box test cut_v2 (Autodesk Fusion 360 design; units mm, degrees)
Autodesk Fusion 360 part; units mm, degrees
note: some values were not read from the file. Set by a fixed rule: which sketch regions a step uses.
sketch "test" plane through (0, 0, 0) normal (0, 0, 1) x (1, 0, 0)
sketch "test (1)" plane through (0, 0, 0) normal (0, 0, 1) x (1, 0, 0)
  line L0 (0, 0) -> (0, 15.1)
  line L1 (0, 15.1) -> (3.175, 15.1)
  line L2 (3.175, 15.1) -> (3.175, 24.9)
  line L3 (3.175, 24.9) -> (0, 24.9)
  line L4 (0, 24.9) -> (0, 35.1)
  line L5 (0, 35.1) -> (3.175, 35.1)
  line L6 (3.175, 35.1) -> (3.175, 44.9)
  line L7 (3.175, 44.9) -> (0, 44.9)
  line L8 (0, 44.9) -> (0, 55.1)
  line L9 (0, 55.1) -> (3.175, 55.1)
  line L10 (3.175, 55.1) -> (3.175, 64.9)
  line L11 (3.175, 64.9) -> (0, 64.9)
  line L12 (0, 64.9) -> (0, 75.1)
  line L13 (0, 75.1) -> (3.175, 75.1)
  line L14 (3.175, 75.1) -> (3.175, 84.9)
  line L15 (3.175, 84.9) -> (0, 84.9)
  line L16 (0, 84.9) -> (0, 95.1)
  line L17 (0, 95.1) -> (3.175, 95.1)
  line L18 (3.175, 95.1) -> (3.175, 104.9)
  line L19 (3.175, 104.9) -> (0, 104.9)
  line L20 (0, 104.9) -> (0, 120)
  circle A0 centre (2.3644, 15.6906) radius 1.005
  circle A1 centre (2.3644, 24.3094) radius 1.005
  circle A2 centre (2.3644, 35.6906) radius 1.005
  circle A3 centre (2.3644, 44.3094) radius 1.005
  circle A4 centre (2.3644, 55.6906) radius 1.005
  circle A5 centre (2.3644, 64.3094) radius 1.005
  circle A6 centre (2.3644, 75.6906) radius 1.005
  circle A7 centre (2.3644, 84.3094) radius 1.005
  circle A8 centre (2.3644, 95.6906) radius 1.005
  circle A9 centre (2.3644, 104.3094) radius 1.005
  line L21 (-5.185, 0) -> (-5.185, 14.9)
  line L22 (-5.185, 14.9) -> (-2.01, 14.9)
  line L23 (-2.01, 14.9) -> (-2.01, 25.1)
  line L24 (-2.01, 25.1) -> (-5.185, 25.1)
  line L25 (-5.185, 25.1) -> (-5.185, 34.9)
  line L26 (-5.185, 34.9) -> (-2.01, 34.9)
  line L27 (-2.01, 34.9) -> (-2.01, 45.1)
  line L28 (-2.01, 45.1) -> (-5.185, 45.1)
  line L29 (-5.185, 45.1) -> (-5.185, 54.9)
  line L30 (-5.185, 54.9) -> (-2.01, 54.9)
  line L31 (-2.01, 54.9) -> (-2.01, 65.1)
  line L32 (-2.01, 65.1) -> (-5.185, 65.1)
  line L33 (-5.185, 65.1) -> (-5.185, 74.9)
  line L34 (-5.185, 74.9) -> (-2.01, 74.9)
  line L35 (-2.01, 74.9) -> (-2.01, 85.1)
  line L36 (-2.01, 85.1) -> (-5.185, 85.1)
  line L37 (-5.185, 85.1) -> (-5.185, 94.9)
  line L38 (-5.185, 94.9) -> (-2.01, 94.9)
  line L39 (-2.01, 94.9) -> (-2.01, 105.1)
  line L40 (-2.01, 105.1) -> (-5.185, 105.1)
  line L41 (-5.185, 105.1) -> (-5.185, 120)
  circle A10 centre (-4.3744, 14.3094) radius 1.005
  circle A11 centre (-4.3744, 25.6906) radius 1.005
  circle A12 centre (-4.3744, 34.3094) radius 1.005
  circle A13 centre (-4.3744, 45.6906) radius 1.005
  circle A14 centre (-4.3744, 54.3094) radius 1.005
  circle A15 centre (-4.3744, 65.6906) radius 1.005
  circle A16 centre (-4.3744, 74.3094) radius 1.005
  circle A17 centre (-4.3744, 85.6906) radius 1.005
  circle A18 centre (-4.3744, 94.3094) radius 1.005
  circle A19 centre (-4.3744, 105.6906) radius 1.005
  line L42 (0, 0) -> (-5.185, 0)
  line L43 (0, 120) -> (-5.185, 120)
  dimension "d13" = 15.1
  dimension "d14" = 3.175
  dimension "d15" = 9.8
  dimension "d16" = 3.175
  dimension "d17" = 10.2
  dimension "d18" = 3.175
  dimension "d19" = 9.8
  dimension "d20" = 3.175
  dimension "d21" = 10.2
  dimension "d22" = 3.175
  dimension "d23" = 9.8
  dimension "d24" = 3.175
  dimension "d25" = 10.2
  dimension "d26" = 3.175
  dimension "d27" = 9.8
  dimension "d28" = 3.175
  dimension "d29" = 10.2
  dimension "d30" = 3.175
  dimension "d31" = 9.8
  dimension "d32" = 3.175
  dimension "d33" = 15.1
  dimension "d34" = 2.01
  dimension "d35" = 2.01
  dimension "d36" = 2.01
  dimension "d37" = 2.01
  dimension "d38" = 2.01
  dimension "d39" = 2.01
  dimension "d40" = 2.01
  dimension "d41" = 2.01
  dimension "d42" = 2.01
  dimension "d43" = 2.01
  dimension "d44" = 14.9
  dimension "d45" = 3.175
  dimension "d46" = 10.2
  dimension "d47" = 3.175
  dimension "d48" = 9.8
  dimension "d49" = 3.175
  dimension "d50" = 10.2
  dimension "d51" = 3.175
  dimension "d52" = 9.8
  dimension "d53" = 3.175
  dimension "d54" = 10.2
  dimension "d55" = 3.175
  dimension "d56" = 9.8
  dimension "d57" = 3.175
  dimension "d58" = 10.2
  dimension "d59" = 3.175
  dimension "d60" = 9.8
  dimension "d61" = 3.175
  dimension "d62" = 10.2
  dimension "d63" = 3.175
  dimension "d64" = 14.9
  dimension "d65" = 2.01
  dimension "d66" = 2.01
  dimension "d67" = 2.01
  dimension "d68" = 2.01
  dimension "d69" = 2.01
  dimension "d70" = 2.01
  dimension "d71" = 2.01
  dimension "d72" = 2.01
  dimension "d73" = 2.01
  dimension "d74" = 2.01
  constraint vertical L0
  constraint horizontal L1
  constraint vertical L2
  constraint horizontal L3
  constraint vertical L4
  constraint horizontal L5
  constraint vertical L6
  constraint horizontal L7
  constraint vertical L8
  constraint horizontal L9
  constraint vertical L10
  constraint horizontal L11
  constraint vertical L12
  constraint horizontal L13
  constraint vertical L14
  constraint horizontal L15
  constraint vertical L16
  constraint horizontal L17
  constraint vertical L18
  constraint horizontal L19
  constraint vertical L20
  constraint vertical L21
  constraint horizontal L22
  constraint vertical L23
  constraint horizontal L24
  constraint vertical L25
  constraint horizontal L26
  constraint vertical L27
  constraint horizontal L28
  constraint vertical L29
  constraint horizontal L30
  constraint vertical L31
  constraint horizontal L32
  constraint vertical L33
  constraint horizontal L34
  constraint vertical L35
  constraint horizontal L36
  constraint vertical L37
  constraint horizontal L38
  constraint vertical L39
  constraint horizontal L40
  constraint vertical L41
  measures "d13" distance of L0.start L0.end
  measures "d14" distance of L0.end L1.end
  measures "d15" distance of L1.end L2.end
  measures "d16" distance of L2.end L3.end
  measures "d17" distance of L3.end L4.end
  measures "d18" distance of L4.end L5.end
  measures "d19" distance of L5.end L6.end
  measures "d20" distance of L6.end L7.end
  measures "d21" distance of L7.end L8.end
  measures "d22" distance of L8.end L9.end
  measures "d23" distance of L9.end L10.end
  measures "d24" distance of L10.end L11.end
  measures "d25" distance of L11.end L12.end
  measures "d26" distance of L12.end L13.end
  measures "d27" distance of L13.end L14.end
  measures "d28" distance of L14.end L15.end
  measures "d29" distance of L15.end L16.end
  measures "d30" distance of L16.end L17.end
  measures "d31" distance of L17.end L18.end
  measures "d32" distance of L18.end L19.end
  measures "d33" distance of L19.end L20.end
  measures "d34" diameter of A0
  measures "d35" diameter of A1
  measures "d36" diameter of A2
  measures "d37" diameter of A3
  measures "d38" diameter of A4
  measures "d39" diameter of A5
  measures "d40" diameter of A6
  measures "d41" diameter of A7
  measures "d42" diameter of A8
  measures "d43" diameter of A9
  measures "d44" distance of L21.start L21.end
  measures "d45" distance of L21.end L22.end
  measures "d46" distance of L22.end L23.end
  measures "d47" distance of L23.end L24.end
  measures "d48" distance of L24.end L25.end
  measures "d49" distance of L25.end L26.end
  measures "d50" distance of L26.end L27.end
  measures "d51" distance of L27.end L28.end
  measures "d52" distance of L28.end L29.end
  measures "d53" distance of L29.end L30.end
  measures "d54" distance of L30.end L31.end
  measures "d55" distance of L31.end L32.end
  measures "d56" distance of L32.end L33.end
  measures "d57" distance of L33.end L34.end
  measures "d58" distance of L34.end L35.end
  measures "d59" distance of L35.end L36.end
  measures "d60" distance of L36.end L37.end
  measures "d61" distance of L37.end L38.end
  measures "d62" distance of L38.end L39.end
  measures "d63" distance of L39.end L40.end
  measures "d64" distance of L40.end L41.end
  measures "d65" diameter of A10
  measures "d66" diameter of A11
  measures "d67" diameter of A12
  measures "d68" diameter of A13
  measures "d69" diameter of A14
  measures "d70" diameter of A15
  measures "d71" diameter of A16
  measures "d72" diameter of A17
  measures "d73" diameter of A18
  measures "d74" diameter of A19
extrude "test (1) body extrude" add sketch "test (1)" along normal blind 3.175 makes body 1
sketch "test (2)" plane through (0, 0, 0) normal (0, 0, 1) x (1, 0, 0)
  line L0 (-10, 0) -> (-10, 14.8)
  line L1 (-10, 14.8) -> (-6.825, 14.8)
  line L2 (-6.825, 14.8) -> (-6.825, 24.6)
  line L3 (-6.825, 24.6) -> (-10, 24.6)
  line L4 (-10, 24.6) -> (-10, 34.8)
  line L5 (-10, 34.8) -> (-6.825, 34.8)
  line L6 (-6.825, 34.8) -> (-6.825, 44.6)
  line L7 (-6.825, 44.6) -> (-10, 44.6)
  line L8 (-10, 44.6) -> (-10, 54.8)
  line L9 (-10, 54.8) -> (-6.825, 54.8)
  line L10 (-6.825, 54.8) -> (-6.825, 64.6)
  line L11 (-6.825, 64.6) -> (-10, 64.6)
  line L12 (-10, 64.6) -> (-10, 74.8)
  line L13 (-10, 74.8) -> (-6.825, 74.8)
  line L14 (-6.825, 74.8) -> (-6.825, 84.6)
  line L15 (-6.825, 84.6) -> (-10, 84.6)
  line L16 (-10, 84.6) -> (-10, 94.8)
  line L17 (-10, 94.8) -> (-6.825, 94.8)
  line L18 (-6.825, 94.8) -> (-6.825, 104.6)
  line L19 (-6.825, 104.6) -> (-10, 104.6)
  line L20 (-10, 104.6) -> (-10, 119.4)
  circle A0 centre (-7.6356, 15.4266) radius 1.005
  circle A1 centre (-7.6356, 23.9734) radius 1.005
  circle A2 centre (-7.6356, 35.4266) radius 1.005
  circle A3 centre (-7.6356, 43.9734) radius 1.005
  circle A4 centre (-7.6356, 55.4266) radius 1.005
  circle A5 centre (-7.6356, 63.9734) radius 1.005
  circle A6 centre (-7.6356, 75.4266) radius 1.005
  circle A7 centre (-7.6356, 83.9734) radius 1.005
  circle A8 centre (-7.6356, 95.4266) radius 1.005
  circle A9 centre (-7.6356, 103.9734) radius 1.005
  line L21 (-15.185, 0) -> (-15.185, 14.66)
  line L22 (-15.185, 14.66) -> (-12.01, 14.66)
  line L23 (-12.01, 14.66) -> (-12.01, 24.86)
  line L24 (-12.01, 24.86) -> (-15.185, 24.86)
  line L25 (-15.185, 24.86) -> (-15.185, 34.66)
  line L26 (-15.185, 34.66) -> (-12.01, 34.66)
  line L27 (-12.01, 34.66) -> (-12.01, 44.86)
  line L28 (-12.01, 44.86) -> (-15.185, 44.86)
  line L29 (-15.185, 44.86) -> (-15.185, 54.66)
  line L30 (-15.185, 54.66) -> (-12.01, 54.66)
  line L31 (-12.01, 54.66) -> (-12.01, 64.86)
  line L32 (-12.01, 64.86) -> (-15.185, 64.86)
  line L33 (-15.185, 64.86) -> (-15.185, 74.66)
  line L34 (-15.185, 74.66) -> (-12.01, 74.66)
  line L35 (-12.01, 74.66) -> (-12.01, 84.86)
  line L36 (-12.01, 84.86) -> (-15.185, 84.86)
  line L37 (-15.185, 84.86) -> (-15.185, 94.66)
  line L38 (-15.185, 94.66) -> (-12.01, 94.66)
  line L39 (-12.01, 94.66) -> (-12.01, 104.86)
  line L40 (-12.01, 104.86) -> (-15.185, 104.86)
  line L41 (-15.185, 104.86) -> (-15.185, 119.52)
  circle A10 centre (-14.3744, 14.0334) radius 1.005
  circle A11 centre (-14.3744, 25.4866) radius 1.005
  circle A12 centre (-14.3744, 34.0334) radius 1.005
  circle A13 centre (-14.3744, 45.4866) radius 1.005
  circle A14 centre (-14.3744, 54.0334) radius 1.005
  circle A15 centre (-14.3744, 65.4866) radius 1.005
  circle A16 centre (-14.3744, 74.0334) radius 1.005
  circle A17 centre (-14.3744, 85.4866) radius 1.005
  circle A18 centre (-14.3744, 94.0334) radius 1.005
  circle A19 centre (-14.3744, 105.4866) radius 1.005
  line L42 (-10, 0) -> (-15.185, 0)
  line L43 (-10, 119.4) -> (-15.185, 119.52)
  dimension "d77" = 14.8
  dimension "d78" = 3.175
  dimension "d79" = 9.8
  dimension "d80" = 3.175
  dimension "d81" = 10.2
  dimension "d82" = 3.175
  dimension "d83" = 9.8
  dimension "d84" = 3.175
  dimension "d85" = 10.2
  dimension "d86" = 3.175
  dimension "d87" = 9.8
  dimension "d88" = 3.175
  dimension "d89" = 10.2
  dimension "d90" = 3.175
  dimension "d91" = 9.8
  dimension "d92" = 3.175
  dimension "d93" = 10.2
  dimension "d94" = 3.175
  dimension "d95" = 9.8
  dimension "d96" = 3.175
  dimension "d97" = 14.8
  dimension "d98" = 2.01
  dimension "d99" = 2.01
  dimension "d100" = 2.01
  dimension "d101" = 2.01
  dimension "d102" = 2.01
  dimension "d103" = 2.01
  dimension "d104" = 2.01
  dimension "d105" = 2.01
  dimension "d106" = 2.01
  dimension "d107" = 2.01
  dimension "d108" = 14.66
  dimension "d109" = 3.175
  dimension "d110" = 10.2
  dimension "d111" = 3.175
  dimension "d112" = 9.8
  dimension "d113" = 3.175
  dimension "d114" = 10.2
  dimension "d115" = 3.175
  dimension "d116" = 9.8
  dimension "d117" = 3.175
  dimension "d118" = 10.2
  dimension "d119" = 3.175
  dimension "d120" = 9.8
  dimension "d121" = 3.175
  dimension "d122" = 10.2
  dimension "d123" = 3.175
  dimension "d124" = 9.8
  dimension "d125" = 3.175
  dimension "d126" = 10.2
  dimension "d127" = 3.175
  dimension "d128" = 14.66
  dimension "d129" = 2.01
  dimension "d130" = 2.01
  dimension "d131" = 2.01
  dimension "d132" = 2.01
  dimension "d133" = 2.01
  dimension "d134" = 2.01
  dimension "d135" = 2.01
  dimension "d136" = 2.01
  dimension "d137" = 2.01
  dimension "d138" = 2.01
  constraint vertical L0
  constraint horizontal L1
  constraint vertical L2
  constraint horizontal L3
  constraint vertical L4
  constraint horizontal L5
  constraint vertical L6
  constraint horizontal L7
  constraint vertical L8
  constraint horizontal L9
  constraint vertical L10
  constraint horizontal L11
  constraint vertical L12
  constraint horizontal L13
  constraint vertical L14
  constraint horizontal L15
  constraint vertical L16
  constraint horizontal L17
  constraint vertical L18
  constraint horizontal L19
  constraint vertical L20
  constraint vertical L21
  constraint horizontal L22
  constraint vertical L23
  constraint horizontal L24
  constraint vertical L25
  constraint horizontal L26
  constraint vertical L27
  constraint horizontal L28
  constraint vertical L29
  constraint horizontal L30
  constraint vertical L31
  constraint horizontal L32
  constraint vertical L33
  constraint horizontal L34
  constraint vertical L35
  constraint horizontal L36
  constraint vertical L37
  constraint horizontal L38
  constraint vertical L39
  constraint horizontal L40
  constraint vertical L41
  measures "d77" distance of L0.start L0.end
  measures "d78" distance of L0.end L1.end
  measures "d79" distance of L1.end L2.end
  measures "d80" distance of L2.end L3.end
  measures "d81" distance of L3.end L4.end
  measures "d82" distance of L4.end L5.end
  measures "d83" distance of L5.end L6.end
  measures "d84" distance of L6.end L7.end
  measures "d85" distance of L7.end L8.end
  measures "d86" distance of L8.end L9.end
  measures "d87" distance of L9.end L10.end
  measures "d88" distance of L10.end L11.end
  measures "d89" distance of L11.end L12.end
  measures "d90" distance of L12.end L13.end
  measures "d91" distance of L13.end L14.end
  measures "d92" distance of L14.end L15.end
  measures "d93" distance of L15.end L16.end
  measures "d94" distance of L16.end L17.end
  measures "d95" distance of L17.end L18.end
  measures "d96" distance of L18.end L19.end
  measures "d97" distance of L19.end L20.end
  measures "d98" diameter of A0
  measures "d99" diameter of A1
  measures "d100" diameter of A2
  measures "d101" diameter of A3
  measures "d102" diameter of A4
  measures "d103" diameter of A5
  measures "d104" diameter of A6
  measures "d105" diameter of A7
  measures "d106" diameter of A8
  measures "d107" diameter of A9
  measures "d108" distance of L21.start L21.end
  measures "d109" distance of L21.end L22.end
  measures "d110" distance of L22.end L23.end
  measures "d111" distance of L23.end L24.end
  measures "d112" distance of L24.end L25.end
  measures "d113" distance of L25.end L26.end
  measures "d114" distance of L26.end L27.end
  measures "d115" distance of L27.end L28.end
  measures "d116" distance of L28.end L29.end
  measures "d117" distance of L29.end L30.end
  measures "d118" distance of L30.end L31.end
  measures "d119" distance of L31.end L32.end
  measures "d120" distance of L32.end L33.end
  measures "d121" distance of L33.end L34.end
  measures "d122" distance of L34.end L35.end
  measures "d123" distance of L35.end L36.end
  measures "d124" distance of L36.end L37.end
  measures "d125" distance of L37.end L38.end
  measures "d126" distance of L38.end L39.end
  measures "d127" distance of L39.end L40.end
  measures "d128" distance of L40.end L41.end
  measures "d129" diameter of A10
  measures "d130" diameter of A11
  measures "d131" diameter of A12
  measures "d132" diameter of A13
  measures "d133" diameter of A14
  measures "d134" diameter of A15
  measures "d135" diameter of A16
  measures "d136" diameter of A17
  measures "d137" diameter of A18
  measures "d138" diameter of A19
extrude "test (2) body extrude" add sketch "test (2)" along normal blind 3.175 separate body makes body 2
sketch "test (3)" plane through (0, 0, 0) normal (0, 0, 1) x (1, 0, 0)
  line L0 (-20, 0) -> (-20, 15.4)
  line L1 (-20, 15.4) -> (-16.825, 15.4)
  line L2 (-16.825, 15.4) -> (-16.825, 25.2)
  line L3 (-16.825, 25.2) -> (-20, 25.2)
  line L4 (-20, 25.2) -> (-20, 35.4)
  line L5 (-20, 35.4) -> (-16.825, 35.4)
  line L6 (-16.825, 35.4) -> (-16.825, 45.2)
  line L7 (-16.825, 45.2) -> (-20, 45.2)
  line L8 (-20, 45.2) -> (-20, 55.4)
  line L9 (-20, 55.4) -> (-16.825, 55.4)
  line L10 (-16.825, 55.4) -> (-16.825, 65.2)
  line L11 (-16.825, 65.2) -> (-20, 65.2)
  line L12 (-20, 65.2) -> (-20, 75.4)
  line L13 (-20, 75.4) -> (-16.825, 75.4)
  line L14 (-16.825, 75.4) -> (-16.825, 85.2)
  line L15 (-16.825, 85.2) -> (-20, 85.2)
  line L16 (-20, 85.2) -> (-20, 95.4)
  line L17 (-20, 95.4) -> (-16.825, 95.4)
  line L18 (-16.825, 95.4) -> (-16.825, 105.2)
  line L19 (-16.825, 105.2) -> (-20, 105.2)
  line L20 (-20, 105.2) -> (-20, 120.6)
  circle A0 centre (-17.6356, 15.9546) radius 1.005
  circle A1 centre (-17.6356, 24.6454) radius 1.005
  circle A2 centre (-17.6356, 35.9546) radius 1.005
  circle A3 centre (-17.6356, 44.6454) radius 1.005
  circle A4 centre (-17.6356, 55.9546) radius 1.005
  circle A5 centre (-17.6356, 64.6454) radius 1.005
  circle A6 centre (-17.6356, 75.9546) radius 1.005
  circle A7 centre (-17.6356, 84.6454) radius 1.005
  circle A8 centre (-17.6356, 95.9546) radius 1.005
  circle A9 centre (-17.6356, 104.6454) radius 1.005
  line L21 (-25.185, 0) -> (-25.185, 15.14)
  line L22 (-25.185, 15.14) -> (-22.01, 15.14)
  line L23 (-22.01, 15.14) -> (-22.01, 25.34)
  line L24 (-22.01, 25.34) -> (-25.185, 25.34)
  line L25 (-25.185, 25.34) -> (-25.185, 35.14)
  line L26 (-25.185, 35.14) -> (-22.01, 35.14)
  line L27 (-22.01, 35.14) -> (-22.01, 45.34)
  line L28 (-22.01, 45.34) -> (-25.185, 45.34)
  line L29 (-25.185, 45.34) -> (-25.185, 55.14)
  line L30 (-25.185, 55.14) -> (-22.01, 55.14)
  line L31 (-22.01, 55.14) -> (-22.01, 65.34)
  line L32 (-22.01, 65.34) -> (-25.185, 65.34)
  line L33 (-25.185, 65.34) -> (-25.185, 75.14)
  line L34 (-25.185, 75.14) -> (-22.01, 75.14)
  line L35 (-22.01, 75.14) -> (-22.01, 85.34)
  line L36 (-22.01, 85.34) -> (-25.185, 85.34)
  line L37 (-25.185, 85.34) -> (-25.185, 95.14)
  line L38 (-25.185, 95.14) -> (-22.01, 95.14)
  line L39 (-22.01, 95.14) -> (-22.01, 105.34)
  line L40 (-22.01, 105.34) -> (-25.185, 105.34)
  line L41 (-25.185, 105.34) -> (-25.185, 120.48)
  circle A10 centre (-24.3744, 14.5854) radius 1.005
  circle A11 centre (-24.3744, 25.8946) radius 1.005
  circle A12 centre (-24.3744, 34.5854) radius 1.005
  circle A13 centre (-24.3744, 45.8946) radius 1.005
  circle A14 centre (-24.3744, 54.5854) radius 1.005
  circle A15 centre (-24.3744, 65.8946) radius 1.005
  circle A16 centre (-24.3744, 74.5854) radius 1.005
  circle A17 centre (-24.3744, 85.8946) radius 1.005
  circle A18 centre (-24.3744, 94.5854) radius 1.005
  circle A19 centre (-24.3744, 105.8946) radius 1.005
  line L42 (-20, 0) -> (-25.185, 0)
  line L43 (-20, 120.6) -> (-25.185, 120.48)
  dimension "d141" = 15.4
  dimension "d142" = 3.175
  dimension "d143" = 9.8
  dimension "d144" = 3.175
  dimension "d145" = 10.2
  dimension "d146" = 3.175
  dimension "d147" = 9.8
  dimension "d148" = 3.175
  dimension "d149" = 10.2
  dimension "d150" = 3.175
  dimension "d151" = 9.8
  dimension "d152" = 3.175
  dimension "d153" = 10.2
  dimension "d154" = 3.175
  dimension "d155" = 9.8
  dimension "d156" = 3.175
  dimension "d157" = 10.2
  dimension "d158" = 3.175
  dimension "d159" = 9.8
  dimension "d160" = 3.175
  dimension "d161" = 15.4
  dimension "d162" = 2.01
  dimension "d163" = 2.01
  dimension "d164" = 2.01
  dimension "d165" = 2.01
  dimension "d166" = 2.01
  dimension "d167" = 2.01
  dimension "d168" = 2.01
  dimension "d169" = 2.01
  dimension "d170" = 2.01
  dimension "d171" = 2.01
  dimension "d172" = 15.14
  dimension "d173" = 3.175
  dimension "d174" = 10.2
  dimension "d175" = 3.175
  dimension "d176" = 9.8
  dimension "d177" = 3.175
  dimension "d178" = 10.2
  dimension "d179" = 3.175
  dimension "d180" = 9.8
  dimension "d181" = 3.175
  dimension "d182" = 10.2
  dimension "d183" = 3.175
  dimension "d184" = 9.8
  dimension "d185" = 3.175
  dimension "d186" = 10.2
  dimension "d187" = 3.175
  dimension "d188" = 9.8
  dimension "d189" = 3.175
  dimension "d190" = 10.2
  dimension "d191" = 3.175
  dimension "d192" = 15.14
  dimension "d193" = 2.01
  dimension "d194" = 2.01
  dimension "d195" = 2.01
  dimension "d196" = 2.01
  dimension "d197" = 2.01
  dimension "d198" = 2.01
  dimension "d199" = 2.01
  dimension "d200" = 2.01
  dimension "d201" = 2.01
  dimension "d202" = 2.01
  constraint vertical L0
  constraint horizontal L1
  constraint vertical L2
  constraint horizontal L3
  constraint vertical L4
  constraint horizontal L5
  constraint vertical L6
  constraint horizontal L7
  constraint vertical L8
  constraint horizontal L9
  constraint vertical L10
  constraint horizontal L11
  constraint vertical L12
  constraint horizontal L13
  constraint vertical L14
  constraint horizontal L15
  constraint vertical L16
  constraint horizontal L17
  constraint vertical L18
  constraint horizontal L19
  constraint vertical L20
  constraint vertical L21
  constraint horizontal L22
  constraint vertical L23
  constraint horizontal L24
  constraint vertical L25
  constraint horizontal L26
  constraint vertical L27
  constraint horizontal L28
  constraint vertical L29
  constraint horizontal L30
  constraint vertical L31
  constraint horizontal L32
  constraint vertical L33
  constraint horizontal L34
  constraint vertical L35
  constraint horizontal L36
  constraint vertical L37
  constraint horizontal L38
  constraint vertical L39
  constraint horizontal L40
  constraint vertical L41
  measures "d141" distance of L0.start L0.end
  measures "d142" distance of L0.end L1.end
  measures "d143" distance of L1.end L2.end
  measures "d144" distance of L2.end L3.end
  measures "d145" distance of L3.end L4.end
  measures "d146" distance of L4.end L5.end
  measures "d147" distance of L5.end L6.end
  measures "d148" distance of L6.end L7.end
  measures "d149" distance of L7.end L8.end
  measures "d150" distance of L8.end L9.end
  measures "d151" distance of L9.end L10.end
  measures "d152" distance of L10.end L11.end
  measures "d153" distance of L11.end L12.end
  measures "d154" distance of L12.end L13.end
  measures "d155" distance of L13.end L14.end
  measures "d156" distance of L14.end L15.end
  measures "d157" distance of L15.end L16.end
  measures "d158" distance of L16.end L17.end
  measures "d159" distance of L17.end L18.end
  measures "d160" distance of L18.end L19.end
  measures "d161" distance of L19.end L20.end
  measures "d162" diameter of A0
  measures "d163" diameter of A1
  measures "d164" diameter of A2
  measures "d165" diameter of A3
  measures "d166" diameter of A4
  measures "d167" diameter of A5
  measures "d168" diameter of A6
  measures "d169" diameter of A7
  measures "d170" diameter of A8
  measures "d171" diameter of A9
  measures "d172" distance of L21.start L21.end
  measures "d173" distance of L21.end L22.end
  measures "d174" distance of L22.end L23.end
  measures "d175" distance of L23.end L24.end
  measures "d176" distance of L24.end L25.end
  measures "d177" distance of L25.end L26.end
  measures "d178" distance of L26.end L27.end
  measures "d179" distance of L27.end L28.end
  measures "d180" distance of L28.end L29.end
  measures "d181" distance of L29.end L30.end
  measures "d182" distance of L30.end L31.end
  measures "d183" distance of L31.end L32.end
  measures "d184" distance of L32.end L33.end
  measures "d185" distance of L33.end L34.end
  measures "d186" distance of L34.end L35.end
  measures "d187" distance of L35.end L36.end
  measures "d188" distance of L36.end L37.end
  measures "d189" distance of L37.end L38.end
  measures "d190" distance of L38.end L39.end
  measures "d191" distance of L39.end L40.end
  measures "d192" distance of L40.end L41.end
  measures "d193" diameter of A10
  measures "d194" diameter of A11
  measures "d195" diameter of A12
  measures "d196" diameter of A13
  measures "d197" diameter of A14
  measures "d198" diameter of A15
  measures "d199" diameter of A16
  measures "d200" diameter of A17
  measures "d201" diameter of A18
  measures "d202" diameter of A19
extrude "test (3) body extrude" add sketch "test (3)" along normal blind 3.175 separate body makes body 3
equation "Version_info = 0 mm" comment "1.1.0 LENGTH 153.0 DEPTH 120.0 HEIGHT 50.0 THICKNESS 3.175 TOOL_DIAMETER 2.01 TOOTH_WIDTH 10.0 KERF -0.1 DELTA_FROM_BOTTOM -0.1 STOCK_X_DIMENSION 304.8 STOCK_Y_DIMENSION 609.6 COMPONENT  REPEATS_L_TMP -1 CREATE_COMPONENTS False CREATE_BODIES 1 CREATE_EMPTY_CONTENTS False CREATE_CONSTRAINTS True CLEAR_PREVIOUSLY_GENERATED_ITEMS True JUST_CLEAR_PREVIOUSLY_GENERATED_ITEMS False CREATE_MANUFACTURING False DEBUG_JUST_ONE_PART False MANUAL_LAYOUT  SKIP_LAYOUT False JUST_BUILD_TEST True DEBUG True"
equation "Length = 153.0 mm" comment "Length (mm)"
equation "Depth = 120.0 mm" comment "Depth (mm)"
equation "Height = 50.0 mm" comment "Height (mm)"
equation "Thickness = 3.175 mm" comment "Thickness (mm)"
equation "Tool_diameter = 2.01 mm" comment "Tool Diameter (mm)"
equation "Tooth_width = 10.0 mm" comment "Target Tooth Width (mm)"
equation "Kerf = -0.1 mm" comment "Kerf (mm)- can be negative"
equation "Delta_from_bottom = -0.1 mm" comment "Additional fine adjustment of bone centers from bottom of holes(mm)- positive makes smaller bottom indents"
equation "Stock_x_dimension = 304.8 mm" comment "Stock X Dimension"
equation "Stock_y_dimension = 609.6 mm" comment "Stock Y Dimension"
equation "Repeats_l_tmp = -1.0 mm" comment "temp hidden"
equation "d14 = Thickness"
equation "d16 = Thickness"
equation "d18 = Thickness"
equation "d20 = Thickness"
equation "d22 = Thickness"
equation "d24 = Thickness"
equation "d26 = Thickness"
equation "d28 = Thickness"
equation "d30 = Thickness"
equation "d32 = Thickness"
equation "d34 = Tool_diameter"
equation "d35 = Tool_diameter"
equation "d36 = Tool_diameter"
equation "d37 = Tool_diameter"
equation "d38 = Tool_diameter"
equation "d39 = Tool_diameter"
equation "d40 = Tool_diameter"
equation "d41 = Tool_diameter"
equation "d42 = Tool_diameter"
equation "d43 = Tool_diameter"
equation "d45 = Thickness"
equation "d47 = Thickness"
equation "d49 = Thickness"
equation "d51 = Thickness"
equation "d53 = Thickness"
equation "d55 = Thickness"
equation "d57 = Thickness"
equation "d59 = Thickness"
equation "d61 = Thickness"
equation "d63 = Thickness"
equation "d65 = Tool_diameter"
equation "d66 = Tool_diameter"
equation "d67 = Tool_diameter"
equation "d68 = Tool_diameter"
equation "d69 = Tool_diameter"
equation "d70 = Tool_diameter"
equation "d71 = Tool_diameter"
equation "d72 = Tool_diameter"
equation "d73 = Tool_diameter"
equation "d74 = Tool_diameter"
equation "d78 = Thickness"
equation "d80 = Thickness"
equation "d82 = Thickness"
equation "d84 = Thickness"
equation "d86 = Thickness"
equation "d88 = Thickness"
equation "d90 = Thickness"
equation "d92 = Thickness"
equation "d94 = Thickness"
equation "d96 = Thickness"
equation "d98 = Tool_diameter"
equation "d99 = Tool_diameter"
equation "d100 = Tool_diameter"
equation "d101 = Tool_diameter"
equation "d102 = Tool_diameter"
equation "d103 = Tool_diameter"
equation "d104 = Tool_diameter"
equation "d105 = Tool_diameter"
equation "d106 = Tool_diameter"
equation "d107 = Tool_diameter"
equation "d109 = Thickness"
equation "d111 = Thickness"
equation "d113 = Thickness"
equation "d115 = Thickness"
equation "d117 = Thickness"
equation "d119 = Thickness"
equation "d121 = Thickness"
equation "d123 = Thickness"
equation "d125 = Thickness"
equation "d127 = Thickness"
equation "d129 = Tool_diameter"
equation "d130 = Tool_diameter"
equation "d131 = Tool_diameter"
equation "d132 = Tool_diameter"
equation "d133 = Tool_diameter"
equation "d134 = Tool_diameter"
equation "d135 = Tool_diameter"
equation "d136 = Tool_diameter"
equation "d137 = Tool_diameter"
equation "d138 = Tool_diameter"
equation "d142 = Thickness"
equation "d144 = Thickness"
equation "d146 = Thickness"
equation "d148 = Thickness"
equation "d150 = Thickness"
equation "d152 = Thickness"
equation "d154 = Thickness"
equation "d156 = Thickness"
equation "d158 = Thickness"
equation "d160 = Thickness"
equation "d162 = Tool_diameter"
equation "d163 = Tool_diameter"
equation "d164 = Tool_diameter"
equation "d165 = Tool_diameter"
equation "d166 = Tool_diameter"
equation "d167 = Tool_diameter"
equation "d168 = Tool_diameter"
equation "d169 = Tool_diameter"
equation "d170 = Tool_diameter"
equation "d171 = Tool_diameter"
equation "d173 = Thickness"
equation "d175 = Thickness"
equation "d177 = Thickness"
equation "d179 = Thickness"
equation "d181 = Thickness"
equation "d183 = Thickness"
equation "d185 = Thickness"
equation "d187 = Thickness"
equation "d189 = Thickness"
equation "d191 = Thickness"
equation "d193 = Tool_diameter"
equation "d194 = Tool_diameter"
equation "d195 = Tool_diameter"
equation "d196 = Tool_diameter"
equation "d197 = Tool_diameter"
equation "d198 = Tool_diameter"
equation "d199 = Tool_diameter"
equation "d200 = Tool_diameter"
equation "d201 = Tool_diameter"
equation "d202 = Tool_diameter"
named bodies: "test (1) body", "test (2) body", "test (3) body"
